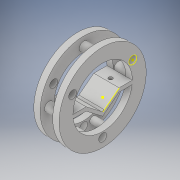
# Autodesk Inventor part: Pen Main Piece
Saved by Autodesk Inventor 2019 (Build 230136000, 136)
## iProperties
Created: 2019-06-10
Part Number: Pen Main Piece
Material: Generic
Document SubType Name: Modeling
Designer: Matthew XPS
Density: 1 g/cm^3
Appearance: Default
Author: Matthew XPS
Autodesk Inventor part; units mm, degrees
ref_plane "YZ Plane" through (0, 0, 0) normal (1, 0, 0) x (0, 1, 0)
ref_plane "XZ Plane" through (0, 0, 0) normal (0, 1, 0) x (-1, 0, 0)
ref_plane "XY Plane" through (0, 0, 0) normal (0, 0, 1) x (1, 0, 0)
sketch "Sketch2" plane through (0, 0, 0) normal (1, 0, 0) x (0, 1, 0)
  circle A0 centre (0, 0) radius 34.5
  circle A1 centre (0, 0) radius 23.5
  dimension "d4" = 69
  dimension "d5" = 11
  constraints: 2 centre point, 1 coincident
  measures "d4" diameter of A0
  measures "d5" radial gap between concentric circles of A0 A1
extrude "Extrusion1" add sketch "Sketch2" along normal blind 5
sketch "Sketch4" plane through (0, 0, 0) normal (1, 0, 0) x (0, 1, 0)
  line L0 (0, 0) -> (-10, 0)
  line L1 (0, -13) -> (-10, 0)
  line L2 (0, -13) -> (0, -24.4889)
  line L3 (0, -13) -> (-3, -13)
  line L4 (-10, 0) -> (-13, 0)
  line L5 (-10, 0) -> (-7, 0) construction
  line L6 (-13, 0) -> (-3, -13)
  line L7 (-3, -13) -> (-3, -25)
  line L8 (0, -24.4889) -> (-3, -25)
  dimension "d16" = 10
  dimension "d17" = 13
  dimension "d18" = 52.431
  dimension "d20" = 3
  dimension "d21" = 3
  dimension "d22" = 180
  dimension "d50" = 12
  constraints: 18 end point, 3 horizontal, 2 vertical, 1 collinear, 1 perpendicular
  measures "d16" distance of L0.start L0.end
  measures "d17" distance of L0.start L1.start
  measures "d18" angle of L0 L1
  measures "d20" distance of L1.start L3.end
  measures "d21" distance of L0.end L4.end
  measures "d22" angle of L4 L5
  measures "d50" distance of L3.end L7.end
extrude "Extrusion2" add sketch "Sketch4" along normal blind 20
mirror "Mirror1" about plane through (0, 0, 0) normal (0, 0, 1) of "Extrusion2"
sketch "Sketch5" plane through (5, 0, 0) normal (1, 0, 0) x (0, 0, -1)
  circle A0 centre (0, 0) radius 23.5 projected
  circle A1 centre (0, 0) radius 34.5 projected
  arc A2 (-23.3077, -3) -> (23.3077, -3) centre (0, 0) ccw projected
  circle A3 centre (0, 0) radius 23.5
  line L0 (-25, -3) -> (-24.4889, 0) projected
  line L1 (-24.4889, 0) -> (-23.5, 0) projected
  arc A4 (23.5, 0) -> (-23.5, 0) centre (0, 0) ccw projected
  line L2 (23.5, 0) -> (24.4889, 0) projected
  line L3 (24.4889, 0) -> (25, -3) projected
  line L4 (-23.3077, -3) -> (-25, -3) projected
  line L5 (25, -3) -> (23.3077, -3) projected
  point P0 (20, 0)
  constraints: 1 centre point, 1 coincident, 1 concentric, 1 other
extrude "Extrusion3" cut sketch "Sketch5" along normal blind 20 contours L2 L3 L5 A0 | A0 L4 L0 L1 | A1
ref_plane "Work Plane1" through (20, 0, 0) normal (-1, 0, 0) x (0, 0, 1)
sketch "Sketch6" plane through (20, 0, 0) normal (-1, 0, 0) x (0, 0, 1)
  arc A0 (23.5, 0) -> (-23.5, 0) centre (0, 0) ccw projected
  circle A1 centre (0, 0) radius 34.5 projected
  arc A2 (-23.5, 0) -> (-23.3077, -3) centre (0, 0) ccw projected
  arc A3 (-23.3077, -3) -> (23.3077, -3) centre (0, 0) ccw projected
  arc A4 (23.3077, -3) -> (23.5, 0) centre (0, 0) ccw projected
extrude "Extrusion4" add sketch "Sketch6" along normal blind 5
sketch "Sketch9" plane through (20, 0, 0) normal (1, 0, 0) x (0, 0, -1)
  circle A0 centre (0, 0) radius 27.5
  circle A1 centre (0, -27.5) radius 3.1
  dimension "d32" = 55
  dimension "d33" = 6.2
  constraints: 1 centre point, 1 coincident, 1 vertical alignment, 2 other
  measures "d33" diameter of A1
extrude "Extrusion5" cut sketch "Sketch9" against normal blind 20 contours A1 A0 | A0 A1 picked at (0.1201, -26.4607) picked at (0.0978, -28.5157)
pattern_circular "Circular Pattern1" count 3 over 360 about axis through (-10, 0, 0) along (1, 0, 0) of "Extrusion5"
sketch "Sketch10" plane through (20, 0, 0) normal (1, 0, 0) x (0, 0, -1)
  circle A0 centre (0, 0) radius 27.5
  circle A1 centre (27.5, 0) radius 3.5
  circle A2 centre (7.328, -26.5057) radius 2.5
  circle A3 centre (-7.328, -26.5057) radius 2.5
  circle A4 centre (-27.5, 0) radius 3.5
  circle A5 centre (0, 27.5) radius 3.5
  dimension "d39" = 55
  dimension "d40" = 7
  dimension "d41" = 5
  dimension "d42" = 5
  dimension "d43" = 7
  dimension "d44" = 7
  constraints: 6 centre point, 5 point on circle, 1 coincident
  measures "d39" diameter of A0
  measures "d40" diameter of A1
  measures "d41" diameter of A2
  measures "d42" diameter of A3
  measures "d43" diameter of A4
  measures "d44" diameter of A5
extrude "Extrusion6" add sketch "Sketch10" against normal blind 20 contours A0 A1 | A0 A1 | A5 A0 | A0 A5 | A2 A0 | A0 A2 | A4 A0 | A0 A4 | A3 A0 | A0 A3
sketch "Sketch11" plane through (0, -3, 13) normal (0, -1, 0) x (1, 0, 0)
  line L0 (0, -36.5) -> (0, 10.5) projected
  line L1 (20, 0) -> (20, 10.3077) projected
  line L2 (20, 5.1539) -> (0, 5.1539)
  line L3 (0, 0) -> (0, 10.3077) projected
  circle A0 centre (10, 5.1539) radius 1.55
  line L4 (10.1694, 5.1539) -> (10.1694, 3.1539)
  line L5 (10.1694, 5.1539) -> (12.1694, 5.1539) construction
  circle A1 centre (10.1694, 3.1539) radius 1.55
  point P0 (0, -13)
  point P1 (20, 9.4891)
  point P2 (0, 9.4891)
  dimension "d47" = 3.1
  dimension "d51" = 2
  dimension "d52" = 90
  dimension "d53" = 3.1
  constraints: 6 end point, 3 midpoint, 2 centre point, 1 coincident, 1 horizontal, 1 parallel, 1 perpendicular, 1 point on line
  measures "d47" diameter of A0
  measures "d51" distance of L4.start L4.end
  measures "d52" angle of L4 L5
  measures "d53" diameter of A1
extrude "Extrusion7" cut sketch "Sketch11" against normal blind 5 contours A1 A0 | A0 L4 A1 | L4 A0 A1
mirror "Mirror2" about plane through (0, 0, 0) normal (0, 0, 1) of "Extrusion7"
sketch "Sketch12" plane through (20, 0, 0) normal (1, 0, 0) x (0, 0, -1)
  line L0 (13, 0) -> (0, -10) projected
sketch "Sketch14" plane through (20, 0, 0) normal (1, 0, 0) x (0, 0, -1)
  circle A0 centre (23.8157, 13.75) radius 3.1 projected
  point P0 (0, 0)
fillet "Fillet1" [suppressed]
fillet "Fillet2" radius 2 1 edges at (10, -10, 0)
body "Solid1"
